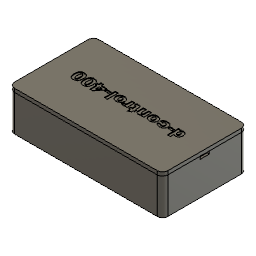
d-control-400-remote-enclosure (Autodesk Fusion 360 design; units mm, degrees)
part number: 2026-07-07-16-35-03-967
Autodesk Fusion 360 part; units mm, degrees
note: some values were not read from the file. Set by a fixed rule: which face or edge a step refers to.
sketch "case" plane through (0, 0, 0) normal (0, 1, 0) x (1, 0, 0)
  line L0 (0, 0) -> (85, 0)
  line L1 (85, 0) -> (85, -46.7)
  line L2 (85, -46.7) -> (0, -46.7)
  line L3 (0, -46.7) -> (0, 0)
  dimension "d1" = 85
  dimension "d2" = 46.7
  constraint horizontal L0
  constraint vertical L1
  constraint horizontal L2
  constraint vertical L3
  constraint coincident L0.start L3.end
  measures "d1" distance of L0.start L0.end
  measures "d2" distance of L0.start L2.end
extrude "Extrude1" add sketch "case" along normal blind 20 makes body 1
shell "Shell1" thickness 2 removed faces 1 at (28.3333, 20, 15.5667) on bodies 1
sketch "standoff" plane through (0, 2, 0) normal (0, 1, 0) x (-1, 0, 0)
  circle A0 centre (-8.85, 41.95) radius 2.75
  line L0 (-78, 2) -> (-2, 2)
  line L1 (-2, 45) -> (-78, 45)
  line L2 (-2, 2) -> (-2, 45)
  line L3 (-2, 45) -> (-78, 45)
  line L4 (-78, 45) -> (-78, 2)
  line L5 (-78, 2) -> (-2, 2)
  line L6 (-2, 44.7) -> (-83, 44.7)
  line L7 (-83, 44.7) -> (-83, 2)
  line L8 (-83, 2) -> (-2, 2)
  line L9 (-2, 2) -> (-2, 44.7)
  dimension "d42" = 5.5
  dimension "d59" = 6.85
  constraint tangent A0 L6
  measures "d42" diameter of A0
  measures "d59" distance of A0.centre L2
extrude "Extrude7" add sketch "standoff" along normal blind 5 contours A0 bodies 1
sketch "standoff_hole" plane through (0, 7, 0) normal (0, 1, 0) x (-1, 0, 0)
  circle A0 centre (-8.85, 41.95) radius 0.9
  circle A1 centre (-8.85, 41.95) radius 2.75
  circle A2 centre (-8.85, 41.95) radius 2.75
  dimension "d47" = 1.8
  constraint concentric A0 A1
  measures "d47" diameter of A0
extrude "Extrude8" cut sketch "standoff_hole" against normal blind 4 contours A0 bodies 1
pattern_linear "R-Pattern3" count 2 spacing 37.2 along (0, 0, -1) of "Extrude7", "Extrude8"
pattern_linear "R-Pattern4" count 2 spacing 45 along (1, 0, 0) of "Extrude7", "Extrude8", "R-Pattern3"
sketch "usb-c_hole" plane through (0, 0, 0) normal (-1, 0, 0) x (0, 0, 1)
  line L0 (0, 0) -> (46.7, 0)
  line L1 (46.7, 0) -> (46.7, 20)
  line L2 (46.7, 20) -> (0, 20)
  line L3 (0, 20) -> (0, 0)
  line L4 (23.35, 20) -> (23.35, 0) construction
  line L5 (20.4338, 9.5) -> (26.2662, 9.5)
  arc A0 (26.2662, 9.5) -> (26.2662, 16.5) centre (26.2662, 13) ccw
  line L6 (26.2662, 16.5) -> (20.4338, 16.5)
  arc A1 (20.4338, 16.5) -> (20.4338, 9.5) centre (20.4338, 13) ccw
  line L7 (20.4338, 13) -> (26.2662, 13) construction
  point P0 (23.35, 13)
  point P1 (16.9338, 13)
  point P2 (29.7662, 13)
  dimension "d63" = 7
  dimension "d64" = 13
  constraint midpoint L2 L4.start
  constraint midpoint L0 L4.end
  constraint tangent L5 A0
  constraint tangent A0 L6
  constraint parallel L5 L6
  constraint tangent L6 A1
  constraint tangent L5 A1
  constraint perpendicular L4 L7
  constraint midpoint L7 P0
  constraint coincident L4 P0
  constraint midpoint A1 P1
  constraint midpoint A0 P2
  measures "d63" diameter of A0
  measures "d64" distance of L0 P0
extrude "Extrude9" cut sketch "usb-c_hole" against normal up to surface (2 mm away) contours L5 A0 L6 A1 bodies 1
sketch "pry_notch" plane through (85, 0, 0) normal (1, 0, 0) x (0, 0, -1)
  line L0 (-46.7, 0) -> (0, 0)
  line L1 (0, 0) -> (0, 20)
  line L2 (0, 20) -> (-46.7, 20)
  line L3 (-46.7, 20) -> (-46.7, 0)
  line L4 (-25.85, 20) -> (-20.85, 20)
  line L5 (-20.85, 20) -> (-20.85, 18.5)
  line L6 (-20.85, 18.5) -> (-25.85, 18.5)
  line L7 (-25.85, 18.5) -> (-25.85, 20)
  dimension "d77" = 5
  dimension "d78" = 1.5
  constraint horizontal L4
  constraint vertical L5
  constraint horizontal L6
  constraint vertical L7
  constraint midpoint L2 L4
  measures "d77" distance of L4.start L4.end
  measures "d78" distance of L4.start L6.end
extrude "Extrude13" cut sketch "pry_notch" against normal blind 1.2 contours L2 L4 L5 L6 L7 bodies 1
fillet "Fillet1" radius 3 4 edges at (85, 10, 0) (85, 10, 46.7) (0, 10, 46.7) (0, 10, 0) on bodies 1
sketch "lid" plane through (0, 20, 0) normal (0, 1, 0) x (-1, 0, 0)
  line L0 (-2, 44.7) -> (-2, 2)
  line L1 (-2, 2) -> (-83, 2)
  line L2 (-83, 2) -> (-83, 44.7)
  line L3 (-83, 44.7) -> (-2, 44.7)
  arc A0 (-3, 0) -> (0, 3) centre (-3, 3) ccw
  line L4 (-3, 0) -> (-82, 0)
  arc A1 (-85, 3) -> (-82, 0) centre (-82, 3) ccw
  line L5 (-85, 3) -> (-85, 43.7)
  arc A2 (-82, 46.7) -> (-85, 43.7) centre (-82, 43.7) ccw
  line L6 (-82, 46.7) -> (-3, 46.7)
  arc A3 (0, 43.7) -> (-3, 46.7) centre (-3, 43.7) ccw
  line L7 (0, 43.7) -> (0, 3)
extrude "Extrude10" add sketch "lid" along normal blind 2 separate body contours L0 L1 L2 L3 | A0 L4 A1 L5 A2 L6 A3 L7 makes body 2
extrude "Extrude11" add sketch "lid" against normal blind 3 contours L0 L1 L2 L3 bodies 2
move_face "OffsetFaces1" offset -0.1 4 faces at (83, 19, 16.2333) (29, 19, 2) (2, 19, 30.4667) (56, 18, 44.7) on bodies 2
chamfer "Chamfer1" distance 0.5 angle 45 4 edges at (42.5, 17, 44.6) (82.9, 17, 23.35) (42.5, 17, 2.1) (2.1, 17, 23.35) tangent chain off on bodies 2
sketch "lid_text" plane through (0, 22, 0) normal (0, 1, 0) x (-1, 0, 0)
  line L0 (-82.4825, 0.8361) -> (-3, 0) construction
  line L1 (-3, 0) -> (-2.5175, 45.8639) construction
  line L2 (-2.5175, 45.8639) -> (-82, 46.7) construction
  line L3 (-82, 46.7) -> (-82.4825, 0.8361) construction
  arc A0 (-82, 46.7) -> (-85, 43.7) centre (-82, 43.7) ccw
  line L4 (-85, 43.7) -> (-85, 3)
  arc A1 (-85, 3) -> (-82, 0) centre (-82, 3) ccw
  line L5 (-82, 0) -> (-3, 0)
  arc A2 (-3, 0) -> (0, 3) centre (-3, 3) ccw
  line L6 (0, 3) -> (0, 43.7)
  arc A3 (0, 43.7) -> (-3, 46.7) centre (-3, 43.7) ccw
  line L7 (-3, 46.7) -> (-82, 46.7)
  dimension "d73" = 6
  dimension "d74" = 0
  text T0 "d-control-400" font "Arial Black" height 6 align centre middle in box 79.4869 x 45.8664 at (-82.4825, 0.8361) x (0.999945, -0.010519) y (0.010519, 0.999945) spacing 1
extrude "Extrude12" cut sketch "lid_text" against normal blind 0.4 text T0 bodies 2
sketch "lid_lip" plane through (0, 17, 0) normal (0, -1, 0) x (1, 0, 0)
  line L0 (2.6, 2.6) -> (82.4, 2.6)
  line L1 (82.4, 2.6) -> (82.4, 44.1)
  line L2 (82.4, 44.1) -> (2.6, 44.1)
  line L3 (2.6, 44.1) -> (2.6, 2.6)
  line L4 (80.4, 42.1) -> (4.6, 42.1)
  line L5 (4.6, 42.1) -> (4.6, 4.6)
  line L6 (4.6, 4.6) -> (80.4, 4.6)
  line L7 (80.4, 4.6) -> (80.4, 42.1)
  dimension "d85" = -2
extrude "Extrude14" cut sketch "lid_lip" against normal blind 3 contours L4 L5 L6 L7 bodies 2
equation "d74 = 'd-control-400'"
named bodies: "case", "lid"
